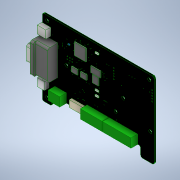
# Autodesk Inventor part: Steering.brd
Saved by Autodesk Inventor 2020 (Build 240168000, 168)
## iProperties
Created: 2019-11-28
Part Number: Steering.brd
Material: Generic
Document SubType Name: Modeling
Designer: kylew
Density: 1 g/cm^3
Appearance: Board Outline
Author: kylew
Autodesk Inventor part; units mm, degrees
ref_plane "YZ Plane" through (0, 0, 0) normal (1, 0, 0) x (0, 1, 0)
ref_plane "XZ Plane" through (0, 0, 0) normal (0, 1, 0) x (-1, 0, 0)
ref_plane "XY Plane" through (0, 0, 0) normal (0, 0, 1) x (1, 0, 0)
sketch "Sketch1" plane through (0, 0, 0) normal (0, 0, 1) x (1, 0, 0)
  line L0 (12, 10) -> (11.4824, 9.9319)
  line L1 (11.4824, 9.9319) -> (11, 9.7321)
  line L2 (11, 9.7321) -> (10.5858, 9.4142)
  line L3 (10.5858, 9.4142) -> (10.2679, 9)
  line L4 (10.2679, 9) -> (10.0681, 8.5176)
  line L5 (10.0681, 8.5176) -> (10, 8)
  line L6 (10, 8) -> (10, 2)
  line L7 (10, 2) -> (9.9319, 1.4824)
  line L8 (9.9319, 1.4824) -> (9.7321, 1)
  line L9 (9.7321, 1) -> (9.4142, 0.5858)
  line L10 (9.4142, 0.5858) -> (9, 0.2679)
  line L11 (9, 0.2679) -> (8.5176, 0.0681)
  line L12 (8.5176, 0.0681) -> (8, 0)
  line L13 (8, 0) -> (2, 0)
  line L14 (2, 0) -> (1.4824, 0.0681)
  line L15 (1.4824, 0.0681) -> (1, 0.2679)
  line L16 (1, 0.2679) -> (0.5858, 0.5858)
  line L17 (0.5858, 0.5858) -> (0.2679, 1)
  line L18 (0.2679, 1) -> (0.0681, 1.4824)
  line L19 (0.0681, 1.4824) -> (0, 2)
  line L20 (0, 2) -> (0, 77)
  line L21 (0, 77) -> (0.0681, 77.5176)
  line L22 (0.0681, 77.5176) -> (0.2679, 78)
  line L23 (0.2679, 78) -> (0.5858, 78.4142)
  line L24 (0.5858, 78.4142) -> (1, 78.7321)
  line L25 (1, 78.7321) -> (1.4824, 78.9319)
  line L26 (1.4824, 78.9319) -> (2, 79)
  line L27 (2, 79) -> (114, 79)
  line L28 (114, 79) -> (114.5176, 78.9319)
  line L29 (114.5176, 78.9319) -> (115, 78.7321)
  line L30 (115, 78.7321) -> (115.4142, 78.4142)
  line L31 (115.4142, 78.4142) -> (115.7321, 78)
  line L32 (115.7321, 78) -> (115.9319, 77.5176)
  line L33 (115.9319, 77.5176) -> (116, 77)
  line L34 (116, 77) -> (116, 2)
  line L35 (116, 2) -> (115.9319, 1.4824)
  line L36 (115.9319, 1.4824) -> (115.7321, 1)
  line L37 (115.7321, 1) -> (115.4142, 0.5858)
  line L38 (115.4142, 0.5858) -> (115, 0.2679)
  line L39 (115, 0.2679) -> (114.5176, 0.0681)
  line L40 (114.5176, 0.0681) -> (114, 0)
  line L41 (114, 0) -> (104, 0)
  line L42 (104, 0) -> (103.4824, 0.0681)
  line L43 (103.4824, 0.0681) -> (103, 0.2679)
  line L44 (103, 0.2679) -> (102.5858, 0.5858)
  line L45 (102.5858, 0.5858) -> (102.2679, 1)
  line L46 (102.2679, 1) -> (102.0681, 1.4824)
  line L47 (102.0681, 1.4824) -> (102, 2)
  line L48 (102, 2) -> (102, 8)
  line L49 (102, 8) -> (101.9319, 8.5176)
  line L50 (101.9319, 8.5176) -> (101.7321, 9)
  line L51 (101.7321, 9) -> (101.4142, 9.4142)
  line L52 (101.4142, 9.4142) -> (101, 9.7321)
  line L53 (101, 9.7321) -> (100.5176, 9.9319)
  line L54 (100.5176, 9.9319) -> (100, 10)
  line L55 (100, 10) -> (12, 10)
  circle A0 centre (2.8, 62.35) radius 0.4
  circle A1 centre (2.8, 69.65) radius 0.4
  circle A2 centre (8.1, 69.65) radius 0.4
  circle A3 centre (8.1, 62.35) radius 0.4
  circle A4 centre (8.97, 48.8) radius 0.595
  circle A5 centre (8.97, 46.51) radius 0.595
  circle A6 centre (8.97, 44.22) radius 0.595
  circle A7 centre (8.97, 41.93) radius 0.595
  circle A8 centre (8.97, 39.64) radius 0.595
  circle A9 centre (11.51, 49.94) radius 0.595
  circle A10 centre (11.51, 47.65) radius 0.595
  circle A11 centre (11.51, 45.36) radius 0.595
  circle A12 centre (11.51, 43.07) radius 0.595
  circle A13 centre (11.51, 40.78) radius 0.595
  circle A14 centre (14.05, 48.8) radius 0.595
  circle A15 centre (14.05, 46.51) radius 0.595
  circle A16 centre (14.05, 44.22) radius 0.595
  circle A17 centre (14.05, 41.93) radius 0.595
  circle A18 centre (14.05, 39.64) radius 0.595
  circle A19 centre (11.51, 31.72) radius 1.59
  circle A20 centre (11.51, 56.72) radius 1.59
  circle A21 centre (72, 18) radius 0.6
  circle A22 centre (75.5, 18) radius 0.6
  circle A23 centre (79, 18) radius 0.6
  circle A24 centre (82.5, 18) radius 0.6
  circle A25 centre (86, 18) radius 0.6
  circle A26 centre (89.5, 18) radius 0.6
  circle A27 centre (93, 18) radius 0.6
  circle A28 centre (96.5, 18) radius 0.6
  circle A29 centre (48.96, 18) radius 0.6
  circle A30 centre (52.46, 18) radius 0.6
  circle A31 centre (55.96, 18) radius 0.6
  circle A32 centre (59.46, 18) radius 0.6
  circle A33 centre (62.96, 18) radius 0.6
  circle A34 centre (66.46, 18) radius 0.6
  circle A35 centre (15.54, 18.02) radius 0.6
  circle A36 centre (19.04, 18.02) radius 0.6
  circle A37 centre (22.54, 18.02) radius 0.6
  circle A38 centre (7.04, 20.74) radius 0.825
  circle A39 centre (7.04, 16.78) radius 0.825
  circle A40 centre (26, 50) radius 0.51
  circle A41 centre (26, 52.54) radius 0.51
  circle A42 centre (28.54, 50) radius 0.51
  circle A43 centre (28.54, 52.54) radius 0.51
  circle A44 centre (31.08, 50) radius 0.51
  circle A45 centre (31.08, 52.54) radius 0.51
  circle A46 centre (105, 63) radius 0.19
  circle A47 centre (111, 63) radius 0.19
  circle A48 centre (114, 56) radius 0.555
  circle A49 centre (114, 58.54) radius 0.555
  circle A50 centre (114, 61.08) radius 0.555
  circle A51 centre (114, 63.62) radius 0.555
  circle A52 centre (114, 66.16) radius 0.555
  circle A53 centre (74, 66.16) radius 0.555
  circle A54 centre (74, 63.62) radius 0.555
  circle A55 centre (74, 61.08) radius 0.555
  circle A56 centre (74, 58.54) radius 0.555
  circle A57 centre (74, 56) radius 0.555
  circle A58 centre (5, 5) radius 1.65
  circle A59 centre (109, 6) radius 1.65
  circle A60 centre (111, 74) radius 1.65
  circle A61 centre (25, 44) radius 1.65
  circle A62 centre (84, 44) radius 1.65
  circle A63 centre (5, 74) radius 1.65
  circle A64 centre (6.1, 64.25) radius 0.45
  circle A65 centre (6.1, 67.75) radius 0.45
  circle A66 centre (113, 27) radius 1.65
  circle A67 centre (75, 27) radius 1.65
  circle A68 centre (23, 58.5) radius 0.1905
  circle A69 centre (37.5, 47) radius 0.1905
  circle A70 centre (46, 47) radius 0.1905
  circle A71 centre (43.5, 71.5) radius 0.1905
  circle A72 centre (48, 74.5) radius 0.1905
  circle A73 centre (50.5, 72) radius 0.1905
  circle A74 centre (67, 53) radius 0.1905
  circle A75 centre (64, 53) radius 0.1905
  circle A76 centre (64, 32) radius 0.1905
  circle A77 centre (64, 28) radius 0.1905
  circle A78 centre (39, 27) radius 0.1905
  circle A79 centre (34, 23) radius 0.1905
  circle A80 centre (47, 73.5) radius 0.1905
  circle A81 centre (49.5, 71) radius 0.1905
  circle A82 centre (67, 66) radius 0.1905
  circle A83 centre (69, 66) radius 0.1905
  circle A84 centre (45, 45) radius 0.1905
  circle A85 centre (42, 43) radius 0.1905
  circle A86 centre (46, 39) radius 0.1905
  circle A87 centre (48.5, 39) radius 0.1905
  circle A88 centre (77, 21.5) radius 0.1905
  circle A89 centre (66, 32) radius 0.1905
  circle A90 centre (48.5, 60) radius 0.1905
  circle A91 centre (17, 58) radius 0.1905
  circle A92 centre (21, 62) radius 0.1905
  circle A93 centre (57.5, 23) radius 0.1905
  circle A94 centre (54.5, 23) radius 0.1905
  circle A95 centre (39.5, 73.5) radius 0.1905
  circle A96 centre (21, 61) radius 0.1905
  circle A97 centre (17, 57) radius 0.1905
  circle A98 centre (35, 72) radius 0.1905
  circle A99 centre (39.1731, 72.25) radius 0.1905
  circle A100 centre (17, 56) radius 0.1905
  circle A101 centre (21, 60) radius 0.1905
  circle A102 centre (15.99, 46.51) radius 0.1905
  circle A103 centre (16, 50) radius 0.1905
  circle A104 centre (34, 71) radius 0.1905
  circle A105 centre (40, 71.5) radius 0.1905
  circle A106 centre (21, 59) radius 0.1905
  circle A107 centre (17, 55) radius 0.1905
  circle A108 centre (64, 56) radius 0.1905
  circle A109 centre (56.5, 61) radius 0.1905
  circle A110 centre (51.5, 67) radius 0.1905
  circle A111 centre (29.25, 41.75) radius 0.1905
  circle A112 centre (41, 41) radius 0.1905
  circle A113 centre (31.5, 39) radius 0.1905
  circle A114 centre (37, 20) radius 0.1905
  circle A115 centre (25, 61) radius 0.1905
  circle A116 centre (96, 67.5) radius 0.1905
  circle A117 centre (93, 67.5) radius 0.1905
  circle A118 centre (90, 67.5) radius 0.1905
  circle A119 centre (10.5, 64) radius 0.1905
  circle A120 centre (54, 52) radius 0.1905
  circle A121 centre (58, 52) radius 0.1905
  circle A122 centre (59, 74) radius 0.1905
  circle A123 centre (62.25, 56.5) radius 0.1905
  circle A124 centre (56.5, 58.5) radius 0.1905
  circle A125 centre (32, 60.8269) radius 0.1905
  circle A126 centre (38, 55) radius 0.1905
  circle A127 centre (35.8269, 52) radius 0.1905
  circle A128 centre (45, 71.5) radius 0.1905
  circle A129 centre (32, 67) radius 0.1905
  circle A130 centre (48, 62.5) radius 0.1905
  circle A131 centre (59, 40.5) radius 0.1905
  circle A132 centre (59, 35.5) radius 0.1905
  circle A133 centre (45, 42.5) radius 0.1905
  circle A134 centre (25.5, 67.75) radius 0.1905
  circle A135 centre (41, 49) radius 0.1905
  circle A136 centre (44, 49) radius 0.1905
  circle A137 centre (42, 22) radius 0.1905
  circle A138 centre (42, 31) radius 0.1905
  circle A139 centre (40, 48) radius 0.1905
  circle A140 centre (43, 48) radius 0.1905
  circle A141 centre (43, 22) radius 0.1905
  circle A142 centre (43, 30) radius 0.1905
  circle A143 centre (28.5, 47.5) radius 0.1905
  circle A144 centre (39, 47) radius 0.1905
  circle A145 centre (32.5, 43) radius 0.1905
  circle A146 centre (54, 45) radius 0.1905
  circle A147 centre (38, 39) radius 0.1905
  circle A148 centre (77, 22.5) radius 0.1905
  circle A149 centre (67, 32) radius 0.1905
  circle A150 centre (43.5, 60.5) radius 0.1905
  circle A151 centre (41.0461, 55.5) radius 0.1905
  circle A152 centre (32.5, 47) radius 0.1905
  circle A153 centre (34.5, 42.5) radius 0.1905
  circle A154 centre (45.5, 58.5) radius 0.1905
  circle A155 centre (54, 56) radius 0.1905
  circle A156 centre (58, 56) radius 0.1905
  circle A157 centre (27.5, 47.5) radius 0.1905
  circle A158 centre (63, 54.5) radius 0.1905
  circle A159 centre (82, 54.5) radius 0.1905
  circle A160 centre (44, 22) radius 0.1905
  circle A161 centre (44, 29) radius 0.1905
  circle A162 centre (35, 56.7493) radius 0.1905
  circle A163 centre (65, 50.5) radius 0.1905
  circle A164 centre (77, 20.5) radius 0.1905
  circle A165 centre (65, 32) radius 0.1905
  line L56 (-263.1716, -325.0539) -> (-15.8331, -325.0539) construction
  line L57 (-15.8331, -325.0539) -> (-15.8331, -489.9462) construction
  line L58 (-15.8331, -489.9462) -> (-263.1716, -489.9462) construction
  line L59 (-263.1716, -489.9462) -> (-263.1716, -325.0539) construction
  constraints: 166 centre point, 112 end point, 2 other
extrude "Steering.brd_Outline" add sketch "Sketch1" along normal blind 1.6
sketch "KINGBRIGHT_LED, LED_AA3528VRVCS_A_1" plane through (0, 0, 1.6) normal (0, 0, 1) x (1, 0, 0)
  line L0 (59.016, 36.8885) -> (55.4525, 36.8885)
  line L1 (55.4525, 36.8885) -> (55.4525, 38.452)
  line L2 (55.4525, 38.452) -> (59.016, 38.452)
  line L3 (59.016, 38.452) -> (59.016, 36.8885)
  constraints: 8 end point
extrude "D2_2" add sketch "KINGBRIGHT_LED, LED_AA3528VRVCS_A_1" along normal blind 1
sketch "KINGBRIGHT_LED, LED_AA3528VRVCS_A_3" plane through (0, 0, 1.6) normal (0, 0, 1) x (1, 0, 0)
  line L0 (59.016, 31.8885) -> (55.4525, 31.8885)
  line L1 (55.4525, 31.8885) -> (55.4525, 33.452)
  line L2 (55.4525, 33.452) -> (59.016, 33.452)
  line L3 (59.016, 33.452) -> (59.016, 31.8885)
  constraints: 8 end point
extrude "D3_4" add sketch "KINGBRIGHT_LED, LED_AA3528VRVCS_A_3" along normal blind 1
sketch "KINGBRIGHT_LED, PINK_5" plane through (0, 0, 1.6) normal (0, 0, 1) x (1, 0, 0)
  line L0 (59.016, 70.3885) -> (55.4525, 70.3885)
  line L1 (55.4525, 70.3885) -> (55.4525, 71.952)
  line L2 (55.4525, 71.952) -> (59.016, 71.952)
  line L3 (59.016, 71.952) -> (59.016, 70.3885)
  constraints: 8 end point
extrude "D4_6" add sketch "KINGBRIGHT_LED, PINK_5" along normal blind 1
sketch "CHIP-LED0603, BLUE_7" plane through (0, 0, 1.6) normal (0, 0, 1) x (1, 0, 0)
  line L0 (27.15, 64.0492) -> (27.15, 64.95)
  line L1 (27.15, 64.95) -> (28.85, 64.95)
  line L2 (28.85, 64.95) -> (28.85, 64.0492)
  line L3 (28.85, 64.0492) -> (27.15, 64.0492)
  constraints: 8 end point
extrude "D7_8" add sketch "CHIP-LED0603, BLUE_7" along normal blind 1
sketch "UX60-MB-5S8, UX60-MB-5S8_9" plane through (0, 0, 1.6) normal (0, 0, 1) x (1, 0, 0)
  line L0 (-0.3017, 70.05) -> (8.7072, 70.05)
  line L1 (8.7072, 70.05) -> (8.7072, 61.95)
  line L2 (8.7072, 61.95) -> (-0.3017, 61.95)
  line L3 (-0.3017, 61.95) -> (-0.3017, 70.05)
  constraints: 8 end point
extrude "J1_10" add sketch "UX60-MB-5S8, UX60-MB-5S8_9" along normal blind 5
sketch "MOLEX_5025850670, MOLEX_5025850670_11" plane through (0, 0, 1.6) normal (0, 0, 1) x (1, 0, 0)
  line L0 (30.4765, 17.1835) -> (44.6035, 17.1835)
  line L1 (44.6035, 17.1835) -> (44.6035, 10.12)
  line L2 (44.6035, 10.12) -> (30.4765, 10.12)
  line L3 (30.4765, 10.12) -> (30.4765, 17.1835)
  constraints: 8 end point
extrude "J3_12" add sketch "MOLEX_5025850670, MOLEX_5025850670_11" along normal blind 2.5
sketch "NONASSMANN_VGA_CONNECTOR, NONASSMANN_VGA_CONNECTOR_13" plane through (0, 0, 1.6) normal (0, 0, 1) x (1, 0, 0)
  line L0 (-6.2135, 28.5765) -> (-6.2135, 59.74)
  line L1 (-6.2135, 59.74) -> (16.2135, 59.74)
  line L2 (16.2135, 59.74) -> (16.2135, 28.5765)
  line L3 (16.2135, 28.5765) -> (-6.2135, 28.5765)
  constraints: 8 end point
extrude "J4_14" add sketch "NONASSMANN_VGA_CONNECTOR, NONASSMANN_VGA_CONNECTOR_13" along normal blind 12.5
sketch "SCREW_TERMINAL_PCB_CONN_8_POLE, PCB_SCREW_TERM_8_15" plane through (0, 0, 1.6) normal (0, 0, 1) x (1, 0, 0)
  line L0 (69.4738, 19.2762) -> (98.95, 19.2762)
  line L1 (98.95, 19.2762) -> (98.95, 9.9238)
  line L2 (98.95, 9.9238) -> (69.4738, 9.9238)
  line L3 (69.4738, 9.9238) -> (69.4738, 19.2762)
  constraints: 8 end point
extrude "J5_16" add sketch "SCREW_TERMINAL_PCB_CONN_8_POLE, PCB_SCREW_TERM_8_15" along normal blind 7
sketch "SCREW_TERMINAL_PCB_CONN_6_POLE, PCB_SCREW_TERM_6_17" plane through (0, 0, 1.6) normal (0, 0, 1) x (1, 0, 0)
  line L0 (46.4338, 19.2762) -> (68.91, 19.2762)
  line L1 (68.91, 19.2762) -> (68.91, 9.9238)
  line L2 (68.91, 9.9238) -> (46.4338, 9.9238)
  line L3 (46.4338, 9.9238) -> (46.4338, 19.2762)
  constraints: 8 end point
extrude "J6_18" add sketch "SCREW_TERMINAL_PCB_CONN_6_POLE, PCB_SCREW_TERM_6_17" along normal blind 7
sketch "SCREW_TERMINAL_PCB_CONN_3_POLE, PCB_SCREW_TERM_3_19" plane through (0, 0, 1.6) normal (0, 0, 1) x (1, 0, 0)
  line L0 (13.0138, 19.2962) -> (24.99, 19.2962)
  line L1 (24.99, 19.2962) -> (24.99, 9.9438)
  line L2 (24.99, 9.9438) -> (13.0138, 9.9438)
  line L3 (13.0138, 9.9438) -> (13.0138, 19.2962)
  constraints: 8 end point
extrude "J7_20" add sketch "SCREW_TERMINAL_PCB_CONN_3_POLE, PCB_SCREW_TERM_3_19" along normal blind 7
sketch "B2PS-CENTERED, B2PS-VH_LF__SN__21" plane through (0, 0, 1.6) normal (0, 0, 1) x (1, 0, 0)
  line L0 (7.14, 22.86) -> (7.14, 14.76)
  line L1 (7.14, 14.76) -> (-0.16, 14.76)
  line L2 (-0.16, 14.76) -> (-0.16, 22.86)
  line L3 (-0.16, 22.86) -> (7.14, 22.86)
  constraints: 8 end point
extrude "J8_22" add sketch "B2PS-CENTERED, B2PS-VH_LF__SN__21" along normal blind 5
sketch "TQFP44, ATMEGA32U4-AU_23" plane through (0, 0, 1.6) normal (0, 0, 1) x (1, 0, 0)
  line L0 (33.8999, 57.8999) -> (33.8999, 70.1001)
  line L1 (33.8999, 70.1001) -> (46.1001, 70.1001)
  line L2 (46.1001, 70.1001) -> (46.1001, 57.8999)
  line L3 (46.1001, 57.8999) -> (33.8999, 57.8999)
  constraints: 8 end point
extrude "MC1_24" add sketch "TQFP44, ATMEGA32U4-AU_23" along normal blind 1
sketch "CTS_DIP_SWITCH, CTS_SWITCH_SPST_25" plane through (0, 0, 1.6) normal (0, 0, 1) x (1, 0, 0)
  line L0 (59.0435, 50.3535) -> (59.0435, 42.67)
  line L1 (59.0435, 42.67) -> (52.8205, 42.67)
  line L2 (52.8205, 42.67) -> (52.8205, 50.3535)
  line L3 (52.8205, 50.3535) -> (59.0435, 50.3535)
  constraints: 8 end point
extrude "S1_26" add sketch "CTS_DIP_SWITCH, CTS_SWITCH_SPST_25" along normal blind 1
sketch "PTS645, PTS645_27" plane through (0, 0, 1.6) normal (0, 0, 1) x (1, 0, 0)
  line L0 (50.9365, 57.0635) -> (61.0635, 57.0635)
  line L1 (61.0635, 57.0635) -> (61.0635, 51)
  line L2 (61.0635, 51) -> (50.9365, 51)
  line L3 (50.9365, 51) -> (50.9365, 57.0635)
  constraints: 8 end point
extrude "U_3_28" add sketch "PTS645, PTS645_27" along normal blind 1
sketch "TSSOP14, CD4066BPWR_29" plane through (0, 0, 1.6) normal (0, 0, 1) x (1, 0, 0)
  line L0 (30.8, 46.55) -> (37.2, 46.55)
  line L1 (37.2, 46.55) -> (37.2, 41.5516)
  line L2 (37.2, 41.5516) -> (30.8, 41.5516)
  line L3 (30.8, 41.5516) -> (30.8, 46.55)
  constraints: 8 end point
extrude "U1_30" add sketch "TSSOP14, CD4066BPWR_29" along normal blind 1
sketch "TSSOP14, CD4066BPWR_31" plane through (0, 0, 1.6) normal (0, 0, 1) x (1, 0, 0)
  line L0 (40.3, 46.55) -> (46.7, 46.55)
  line L1 (46.7, 46.55) -> (46.7, 41.5516)
  line L2 (46.7, 41.5516) -> (40.3, 41.5516)
  line L3 (40.3, 41.5516) -> (40.3, 46.55)
  constraints: 8 end point
extrude "U2_32" add sketch "TSSOP14, CD4066BPWR_31" along normal blind 1
sketch "Sketch18" plane through (0, 0, 14.1) normal (0, 0, 1) x (1, 0, 0)
  line L0 (16.2135, 59.74) -> (16.2135, 28.5765) projected
  line L1 (16.2135, 28.5765) -> (0, 28.5765) projected
  line L2 (16.2135, 59.74) -> (3.2135, 59.74)
  line L3 (3.2135, 59.74) -> (3.2135, 28.5765)
  line L4 (3.2135, 28.5765) -> (16.2135, 28.5765)
  line L5 (16.2135, 28.5765) -> (16.2135, 59.74)
  point P0 (0, 0)
  dimension "d42" = 13
  constraints: 8 end point, 2 parallel, 1 horizontal, 1 perpendicular, 1 point on line
  measures "d42" distance of L4.end L3.end
extrude "Extrusion18" cut sketch "Sketch18" against normal blind 2
sketch "Sketch19" plane through (-6.2135, 28.5765, 1.6) normal (-1, 0, 0) x (0, 0, 1)
  line L0 (12.5, 31.1635) -> (12.5, 0) projected
  line L1 (0, 0) -> (10.5, 0) projected
  line L2 (12.5, 31.1635) -> (0, 31.1635)
  line L3 (0, 31.1635) -> (0, 0)
  line L4 (0, 0) -> (12.5, 0)
  line L5 (12.5, 0) -> (12.5, 31.1635)
  line L6 (4.25, 23.8317) -> (8.25, 23.8317)
  line L7 (10.25, 21.8317) -> (10.25, 9.3317)
  line L8 (8.25, 7.3317) -> (4.25, 7.3317)
  line L9 (2.25, 9.3317) -> (2.25, 21.8317)
  line L10 (2.25, 23.8317) -> (10.25, 7.3317) construction
  line L11 (10.25, 23.8317) -> (2.25, 7.3317) construction
  arc A0 (4.25, 23.8317) -> (2.25, 21.8317) centre (4.25, 21.8317) ccw
  arc A1 (2.25, 9.3317) -> (4.25, 7.3317) centre (4.25, 9.3317) ccw
  arc A2 (8.25, 7.3317) -> (10.25, 9.3317) centre (8.25, 9.3317) ccw
  arc A3 (10.25, 21.8317) -> (8.25, 23.8317) centre (8.25, 21.8317) ccw
  point P0 (-1.6, -28.5765)
  point P1 (6.25, 15.5817)
  point P2 (12.5, 0)
  dimension "d45" = 8
  dimension "d46" = 16.5
  dimension "d47" = 15.5817
  dimension "d48" = 6.25
  dimension "d49" = 2
  constraints: 20 end point, 8 point on circle, 8 point on line, 8 tangent, 4 centre point, 4 parallel, 3 equal radius, 2 horizontal, 2 midpoint, 2 perpendicular
  measures "d45" distance of L10.end L11.end
  measures "d46" distance of L11.start L10.end
  measures "d47" distance from line of L1 point (6.25, 15.582)
  measures "d48" distance from line of L0 point (6.25, 15.582)
  measures "d49" radius of A0
extrude "Extrusion19" cut sketch "Sketch19" against normal blind 6
fillet "Fillet1" radius 2 4 edges at (1.5, 28.5765, 14.1) (1.5, 59.74, 14.1) (9.7135, 28.5765, 12.1) (9.7135, 59.74, 12.1)
sketch "Patchwork_Repair" plane through (0, 0, 1.6) normal (0, 0, 1) x (1, 0, 0)
  line L0 (71.5391, 30.9526) -> (115.5391, 30.9526)
  line L1 (115.5391, 30.9526) -> (115.5391, 21.9526)
  line L2 (115.5391, 21.9526) -> (71.5391, 21.9526)
  line L3 (71.5391, 21.9526) -> (71.5391, 30.9526)
  line L4 (116, 2) -> (116, 77) projected
  line L5 (114, 79) -> (2, 79) projected
  line L6 (115.5391, 21.9526) -> (105.5391, 21.9526)
  line L7 (105.5391, 21.9526) -> (105.5391, 2.4526)
  line L8 (105.5391, 2.4526) -> (115.5391, 2.4526)
  line L9 (115.5391, 2.4526) -> (115.5391, 21.9526)
  point P0 (0, 0)
  dimension "d54" = 44
  dimension "d55" = 9
  dimension "d56" = 0.4609
  dimension "d57" = 57.0474
  dimension "d68" = 10
  dimension "d69" = 19.5
  constraints: 16 end point, 4 parallel, 2 horizontal, 2 perpendicular
  measures "d54" distance of L1.end L2.end
  measures "d55" distance of L0.end L1.end
  measures "d56" distance between parallel lines of L4 L1
  measures "d57" distance between parallel lines of L5 L2
  measures "d68" distance of L8.end L7.end
  measures "d69" distance of L7.end L6.end
extrude "Hole Fixing" add sketch "Patchwork_Repair" against normal up to surface (1.6 mm away)
sketch "Sketch21" plane through (0, 0, 1.6) normal (0, 0, 1) x (1, 0, 0)
  circle A0 centre (76, 28) radius 1.65
  circle A1 centre (112, 28) radius 1.65
  line L0 (104, 0) -> (114, 0) projected
  line L1 (0, 28.5765) -> (0, 22.86) projected
  circle A2 centre (109, 5) radius 1.65
  line L2 (102, 8) -> (102, 2) projected
  point P0 (0, 0)
  dimension "d60" = 3.3
  dimension "d61" = 3.3
  dimension "d62" = 28
  dimension "d63" = 28
  dimension "d64" = 36
  dimension "d65" = 76
  dimension "d70" = 3.3
  dimension "d71" = 7
  dimension "d72" = 5
  constraints: 3 centre point
  measures "d60" diameter of A0
  measures "d61" diameter of A1
  measures "d62" distance from line of L0 A0.centre
  measures "d63" distance from line of L0 A1.centre
  measures "d64" distance of A1.centre A0.centre
  measures "d65" distance from line of L1 A0.centre
  measures "d70" diameter of A2
  measures "d71" distance from line of L2 A2.centre
  measures "d72" distance from line of L0 A2.centre
extrude "Extrusion21" cut sketch "Sketch21" against normal through all contours A0 | A1
body "Solid1"
